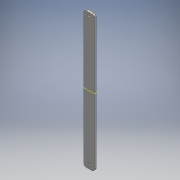
# Autodesk Inventor part: pin
Saved by Autodesk Inventor 2016 (Build 200138000, 138)
## iProperties
Created: 2018-10-08
Part Number: pin
Material: Generic
Document SubType Name: Modeling
Designer: andrew
Density: 1 g/cm^3
Appearance: Default
Author: andrew
Autodesk Inventor part; units mm, degrees
ref_plane "YZ Plane" through (0, 0, 0) normal (1, 0, 0) x (0, 1, 0)
ref_plane "XZ Plane" through (0, 0, 0) normal (0, 1, 0) x (-1, 0, 0)
ref_plane "XY Plane" through (0, 0, 0) normal (0, 0, 1) x (1, 0, 0)
sketch "Sketch1" plane through (0, 0, 0) normal (0, 1, 0) x (-1, 0, 0)
  line L0 (-7.5, 100) -> (7.5, 100)
  line L1 (7.5, 100) -> (7.5, -100)
  line L2 (7.5, -100) -> (-7.5, -100)
  line L3 (-7.5, -100) -> (-7.5, 100)
  line L4 (-7.5, 100) -> (7.5, -100) construction
  line L5 (7.5, 100) -> (-7.5, -100) construction
  point P0 (0, 0)
  dimension "d0" = 15
  dimension "d1" = 200
  constraints: 12 end point, 2 midpoint, 2 parallel, 1 horizontal, 1 perpendicular
  measures "d0" distance of L1.end L2.end
  measures "d1" distance of L0.end L1.end
extrude "Extrusion1" add sketch "Sketch1" along normal blind 3
sketch "Sketch2" plane through (0, 3, 0) normal (0, 1, 0) x (1, 0, 0)
  line L0 (7.5, 100) -> (-7.5, 100) construction
  line L1 (0, 100) -> (0, 95) construction
  point P0 (0, 0)
  dimension "d4" = 5
  constraints: 2 end point, 1 midpoint, 1 vertical
  measures "d4" distance of L1.start L1.end
hole "Hole1" at (0, 3, -95) direction (0, -1, 0) diameter 3 end through all
ref_plane "Work Plane1" through (-7.5, 0, 0) normal (0, 0, 1) x (1, 0, 0)
mirror "Mirror1" about plane through (-7.5, 0, 0) normal (0, 0, 1) of "Hole1"
fillet "Fillet1" radius 3 4 edges at (7.5, 1.5, -100) (-7.5, 1.5, -100) (7.5, 1.5, 100) (-7.5, 1.5, 100)
body "Solid1"
